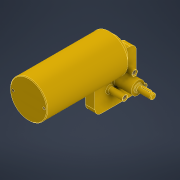
# Autodesk Inventor part: motor
Saved by Autodesk Inventor 2021 (Build 250183000, 183)
## iProperties
Created: 2021-06-20
Part Number: motor
Material: Generic
Document SubType Name: Modeling
Designer: Watchdog
Density: 2.77592 g/cm^3
Appearance: Gold
Mass: 1250 g
Surface Area: 425.35 cm^2
Volume: 450.301 cm^3
Author: Watchdog
Autodesk Inventor part; units mm, degrees
ref_plane "XY Plane" through (0, 0, 0) normal (0, 0, 1) x (1, 0, 0)
sketch "Sketch1" plane through (0, 0, 0) normal (0, 0, 1) x (1, 0, 0)
  circle A0 centre (0, 0) radius 30
  dimension "d0" = 60
  constraints: 1 centre point, 1 coincident
  measures "d0" diameter of A0
extrude "Extrusion1" add sketch "Sketch1" along normal blind 139
ref_plane "Work Plane1" through (62, 0, 0) normal (1, 0, 0) x (0, 1, 0)
ref_plane "Work Plane2" through (0, 0, 0) normal (1, 0, 0) x (0, 1, 0)
sketch "Sketch2" plane through (0, 0, 0) normal (1, 0, 0) x (0, 1, 0)
  point P0 (0, 0)
ref_plane "Work Plane3" through (0, 0, 0) normal (0, 0, -1) x (-1, 0, 0)
sketch "Sketch3" plane through (0, 0, 0) normal (0, 0, -1) x (-1, 0, 0)
  line L0 (0, -34.6) -> (-62, -34.6)
  line L1 (-62, -34.6) -> (-62, -30.1)
  line L2 (-62, -30.1) -> (-40, -30.1)
  line L3 (-40, -30.1) -> (-40, -29.1)
  line L4 (-40, -29.1) -> (-38, -29.1)
  line L5 (-38, -29.1) -> (-38, -28.1)
  line L6 (-38, -28.1) -> (-37, -28.1)
  line L7 (-37, -28.1) -> (-37, -24.1)
  line L8 (-37, -24.1) -> (0, -24.1)
  line L9 (0, -24.1) -> (0, -34.6)
  point P0 (0, 0)
  dimension "d6" = 62
  dimension "d7" = 34.6
  dimension "d15" = 4.5
  dimension "d16" = 22
  dimension "d17" = 1
  dimension "d18" = 2
  dimension "d19" = 1
  dimension "d20" = 1
  dimension "d21" = 4
  dimension "d22" = 0
  constraints: 20 end point, 6 perpendicular, 3 vertical, 1 horizontal
  measures "d6" distance of L0.start L0.end
  measures "d7" distance from line of point (0, 0) L0
  measures "d15" distance of L0.end L1.end
  measures "d16" distance of L1.end L2.end
  measures "d17" distance of L2.end L3.end
  measures "d18" distance of L3.end L4.end
  measures "d19" distance of L4.end L5.end
  measures "d20" distance of L5.end L6.end
  measures "d21" distance of L6.end L7.end
  measures "d22" distance from line of point (0, 0) L9
sketch "Sketch4" plane through (0, 0, 0) normal (1, 0, 0) x (0, 1, 0)
  line L0 (-30, 0) -> (-30, 139) projected
  line L1 (0, 39.5) -> (-70.6, 39.5)
  line L2 (-70.6, -27) -> (0, -27)
  line L3 (0, -27) -> (0, 39.5)
  line L4 (-70.6, 39.5) -> (-70.6, -27)
  line L5 (30, 0) -> (30, 139) projected
  point P0 (0, 0)
  point P1 (-30, 39.5)
  dimension "d11" = 0
  dimension "d12" = 99.5
  dimension "d13" = 66.5
  dimension "d14" = 100.6
  constraints: 8 end point, 1 horizontal, 1 parallel, 1 vertical
  measures "d11" distance from line of point (0, 0) L3
  measures "d12" distance from line of L1 point (-30, 139)
  measures "d13" distance between parallel lines of L1 L2
  measures "d14" distance between parallel lines of L4 L5
extrude "Extrusion2" add sketch "Sketch4" along normal mid plane 15
revolve "Revolution1" add sketch "Sketch3" angle 360 about axis through (0, -34.6, 0) along (1, 0, 0)
ref_plane "Work Plane4" through (51, -30.1, 0) normal (0, 1, 0) x (-1, 0, 0)
sketch "Sketch5" plane through (51, -30.1, 0) normal (0, 1, 0) x (-1, 0, 0)
  line L0 (-11, -4.5) -> (-11, 4.5) projected
  line L1 (99.4, 0) -> (-29.4, 0) projected
  line L2 (6.5, 0) -> (-6.5, 0) construction
  line L3 (6.5, 1.5) -> (-6.5, 1.5)
  line L4 (-6.5, -1.5) -> (6.5, -1.5)
  arc A0 (6.5, -1.5) -> (6.5, 1.5) centre (6.5, 0) ccw
  arc A1 (-6.5, 1.5) -> (-6.5, -1.5) centre (-6.5, 0) ccw
  point P0 (51, 0)
  point P1 (0, 0)
  dimension "d28" = 3
  dimension "d29" = 0
  dimension "d30" = 13
  dimension "d31" = 4.5
  constraints: 8 end point, 4 point on circle, 4 tangent, 2 centre point, 1 horizontal, 1 midpoint, 1 parallel
  measures "d28" distance between parallel lines of L4 L3
  measures "d29" distance from line of L1 point (0, 0)
  measures "d30" distance of L2.end L2.start
  measures "d31" distance from line of L0 L2.end
extrude "Extrusion3" add sketch "Sketch5" against normal up to surface round surface about axis through (51, -34.6, 0) along (-1, 0, 0) radius 4.5 far side no
sketch "Sketch6" plane through (51, -30.1, 0) normal (0, 1, 0) x (1, 0, 0)
  arc A0 (-8, 0) -> (-6.5, -1.5) centre (-6.5, 0) ccw projected
  line L0 (-6.5, -1.5) -> (6.5, -1.5) projected
  arc A1 (6.5, -1.5) -> (8, 0) centre (6.5, 0) ccw projected
  arc A2 (8, 0) -> (6.5, 1.5) centre (6.5, 0) ccw projected
  line L1 (6.5, 1.5) -> (-6.5, 1.5) projected
  arc A3 (-6.5, 1.5) -> (-8, 0) centre (-6.5, 0) ccw projected
  point P0 (-51, 0)
extrude "Extrusion4" add sketch "Sketch6" along normal blind 1.3
chamfer "Chamfer1" distance 1 angle 45 1 edges at (62, -39.1, 0)
fillet "Fillet1" radius 10 3 edges at (0, 0, -27) (0, -70.6, -27) (0, -70.6, 39.5)
sketch "Sketch7" plane through (0, 0, 139) normal (0, 0, 1) x (1, 0, 0)
  point P0 (0, 0)
  point P1 (0, 0)
  point P2 (-25, 0)
  point P3 (25, 0)
  dimension "d42" = 0
  dimension "d43" = 0
  dimension "d44" = 25
  dimension "d45" = 25
  measures "d42" vertical distance of point (0, 0) point (25, 0)
  measures "d43" vertical distance of point (0, 0) point (-25, 0)
  measures "d44" distance of point (0, 0) point (-25, 0)
  measures "d45" distance of point (0, 0) point (25, 0)
hole "Hole1" at (-25, 0, 139) at (25, 0, 139) direction (0, 0, -1) diameter 4.134 depth 8 tip angle 118 thread size "M5x0.8" class "6H" standard "ISO Metric profile"
chamfer "Chamfer3" distance 9 angle 45 2 edges at (-18.3712, 23.7171, 0) (26.7953, -13.4912, 0)
chamfer "Chamfer4" distance 1 angle 45 1 edges at (-30, 0, 139)
ref_plane "Work Plane5" through (32, -34.6, 0) normal (1, 0, 0) x (0, 0, -1)
sketch "Sketch8" plane through (32, -34.6, 0) normal (1, 0, 0) x (0, 0, -1)
  circle A0 centre (0, 0) radius 18
  circle A1 centre (0, 0) radius 3.5 projected
  circle A2 centre (0, 0) radius 10.5 projected
  line L0 (0, 0) -> (-15.5885, -9)
  line L1 (0, 0) -> (15.5885, -9)
  line L2 (0, 0) -> (0, 18)
  circle A3 centre (-15.5885, -9) radius 3
  circle A4 centre (-15.5885, -9) radius 4.5
  circle A5 centre (15.5885, -9) radius 3
  circle A6 centre (15.5885, -9) radius 4.5
  circle A7 centre (0, 18) radius 3
  circle A8 centre (0, 18) radius 4.5
  point P0 (0, 34.6)
  dimension "d64" = 36
  dimension "d67" = 120
  dimension "d68" = 120
  dimension "d69" = 6
  dimension "d70" = 9
  dimension "d71" = 6
  dimension "d72" = 9
  dimension "d73" = 6
  dimension "d74" = 9
  constraints: 9 coincident, 7 centre point, 6 end point, 3 point on circle, 1 concentric, 1 vertical
  measures "d64" diameter of A0
  measures "d67" angle of L0 L2
  measures "d68" angle of L1 L2
  measures "d69" diameter of A3
  measures "d70" diameter of A4
  measures "d71" diameter of A5
  measures "d72" diameter of A6
  measures "d73" diameter of A7
  measures "d74" diameter of A8
extrude "Extrusion5" add sketch "Sketch8" against normal up to next contours A8 L2 A7 A0 | A0 A7 A8 | A6 A0 A5 | A0 A5 L1 A6 | A8 A0 A7 L2 | L1 A5 A0 A6 | A4 L0 A3 A0 | A0 A3 A4 | A0 A3 L0 A4
chamfer "Chamfer5" distance 2 angle 45 11 edges at (7.5, -43.6, 20.0885) (7.5, -43.6992, -5.2396) (7.5, -28.9101, 8.8247) (7.5, -24.6074, 3.2246) (7.5, -29.2666, 9.0446) (7.5, -24.1004, -0.0919) (7.5, -43.6, -11.0885) (7.5, -19.6685, -3.2916) (7.5, -13.418, -3.182) (7.5, -21.0972, -0.1577) (7.5, -21.0568, 0.6217)
sketch "Sketch9" plane through (32, -16.6, 0) normal (1, 0, 0) x (0, 0, -1)
  line L0 (0, -3) -> (0, 3) projected
  circle A0 centre (0, 0) radius 3
  point P0 (0, 16.6)
  dimension "d80" = 6
  constraints: 1 centre point, 1 midpoint
  measures "d80" diameter of A0
extrude "Extrusion6" cut sketch "Sketch9" against normal up to surface (24.5 mm away)
thread "Thread1" size "M6x1" class "6H" standard "ISO Metric profile" full length
thread "Thread2" size "M6x1" class "6H" standard "ANSI Metric M Profile" full length
thread "Thread3" size "M6x1" class "6H" standard "ANSI Metric M Profile" full length
chamfer "Chamfer6" distance 1 angle 45 3 edges at (32, -16.6, 3) (32, -43.6, 18.5885) (32, -43.6, -12.5885)
ref_plane "calibration32" through (32, 0, 0) normal (1, 0, 0) x (0, 1, 0)
body "Solid1"
